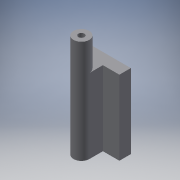
# Autodesk Inventor part: connector9V
Saved by Autodesk Inventor 2018 (Build 220112000, 112)
## iProperties
Created: 2018-07-19
Part Number: connector9V
Material: Generic
Document SubType Name: Modeling
Designer: julien.allali
Density: 1 g/cm^3
Appearance: Default
Author: julien.allali
Autodesk Inventor part; units mm, degrees
ref_plane "YZ Plane" through (0, 0, 0) normal (1, 0, 0) x (0, 1, 0)
ref_plane "XZ Plane" through (0, 0, 0) normal (0, 1, 0) x (-1, 0, 0)
ref_plane "XY Plane" through (0, 0, 0) normal (0, 0, 1) x (1, 0, 0)
sketch "Sketch1" plane through (0, 0, 0) normal (0, 0, 1) x (1, 0, 0)
  circle A0 centre (0, -7.5) radius 2.8 projected
  line L0 (-2.2805, 10.95) -> (2.2805, 10.95) projected
  line L1 (2.2805, 10.95) -> (4.5611, 7) projected
  line L2 (4.5611, 7) -> (2.2805, 3.05) projected
  line L3 (2.2805, 3.05) -> (-2.2805, 3.05) projected
  line L4 (-2.2805, 3.05) -> (-4.5611, 7) projected
  line L5 (-4.5611, 7) -> (-2.2805, 10.95) projected
  line L6 (8.5, 13) -> (-8.5, 13) projected
  line L7 (-8.5, 13) -> (-8.5, -13) projected
  line L8 (-8.5, -13) -> (8.5, -13) projected
  line L9 (8.5, -13) -> (8.5, 13) projected
  point P0 (0, 0)
extrude "Extrusion1" add sketch "Sketch1" along normal blind 2
sketch "Sketch2" plane through (0, 0, 2) normal (0, 0, 1) x (1, 0, 0)
  line L0 (8.5, -13) -> (8.5, 13) projected
  line L1 (8.5, 13) -> (-8.5, 13) projected
  line L2 (-8.5, 13) -> (-8.5, -13) projected
  line L3 (-8.5, -13) -> (8.5, -13) projected
  point P0 (0, 0)
extrude "Extrusion2" add sketch "Sketch2" along normal blind 2
sketch "Sketch3" plane through (-8.5, 13, 0) normal (0, 1, 0) x (1, 0, 0)
  circle A0 centre (8.5, -8.75) radius 2.75
  circle A1 centre (8.5, -8.75) radius 1.05
  line L0 (0, -4) -> (17, -4) construction
  line L1 (8.5, -4) -> (8.5, -22.1376) construction
  point P0 (8.5, 0)
  dimension "d4" = 5.5
  dimension "d5" = 2.1
  dimension "d6" = 4.75
  constraints: 2 centre point, 2 end point, 1 coincident, 1 midpoint, 1 point on line, 1 vertical
  measures "d4" diameter of A0
  measures "d5" diameter of A1
  measures "d6" distance from line of L0 A0.centre
extrude "Extrusion3" add sketch "Sketch3" along normal blind 10
sketch "Sketch4" plane through (0, 13, 8.75) normal (0, -1, 0) x (1, 0, 0)
  circle A0 centre (0, 0) radius 2.75 projected
  line L0 (-2.75, 0) -> (2.75, 0)
  line L1 (2.75, 0) -> (2.75, -4.75)
  line L2 (2.75, -4.75) -> (-2.75, -4.75)
  line L3 (-2.75, -4.75) -> (-2.75, 0)
  line L4 (-8.5, -4.75) -> (8.5, -4.75) projected
  point P0 (0, -8.75)
  constraints: 8 end point, 2 parallel, 2 tangent, 1 collinear, 1 horizontal, 1 midpoint, 1 perpendicular
extrude "Extrusion4" add sketch "Sketch4" along normal up to surface (26 mm away)
body "Solid1"
